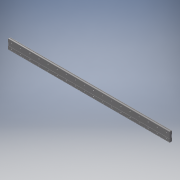
# Autodesk Inventor part: LWLF42...BCSR710Track Rail
Saved by Autodesk Inventor 2016 (Build 200138000, 138)
## iProperties
Category: PARTsolutions
Company: IKO
Created: 2015-04-20
Part Number: LWLF42...BCSR710Track Rail
Catalog Web Link: www.cadenas.de
Description: LWLF Track-LWLF
Vendor: IKO
Document SubType Name: Modeling
Designer: PARTuser1
Manufacturer: IKO
Mass: 2162.88 g
Surface Area: 840.251 cm^2
Volume: 270.361 cm^3
Density: 8 g/cm^3
Material: Stainless Steel
Appearance: Semi-Polished
PSOL_IDENT_0: {$CADENAS_DATA\23d-libs\iko\linear_way_series\linear_way_l_series\lwlf\lwlf4\lwlf_track.prj},207 {VT
PSOL_IDENT_1: YP=3D},{NB=LWLF42...BCSR710Track Rail},{LINA=LWLF42...BCSR710Track Rail},{NN=LWLF Track},{DATE=11.12
PSOL_IDENT_2: .2014 01:21:34},{GEOMDATE=16.10.2008 00:00:00},{VERSION=},{LINEID=230},{LINESUBID=-1},{WBVAR=L,SP,RE
PSOL_IDENT_3: F}  {NB=LWLF42...BCSR710Track Rail},{LINA=LWLF42...BCSR710Track Rail},{KT=DUMMY},{MN=LWLF42},{MNX=LW
PSOL_IDENT_4: LF42...BCS},{L=710.00},{SP=},{REF=},{W=42.000},{H4=10.000},{D3=4.500},{D4=8.000},{HM=4.500},{E1=15},
PSOL_IDENT_5: {E2=15},{F=40.000},{H1=4.000},{L1D=1075.00},{NX=1},{N=1},{N1=1},{P=18},{SP1='', 'No', 'S', 'Yes'},{P
PSOL_IDENT_6: 1D=53},{LS=1520.000},{LMAX=1600.000},{LX=680},{LY=1520},{LZ=1560},{PS=38},{LMINS=67},{EK=30},{EMIN=6
PSOL_IDENT_7: .500},{EMINJ=6.500},{EMAXJ=26.500},{PV=110},{P1D1=55},{EMIND=6.5},{LV=2230},{ED=20},{ED1=0},{L1=54.8
PSOL_IDENT_8: 00},{L4=60.000},{A=2.500},{C=2.000},{LMIN=60.00},{LEND=1560.00},{RK=1.50},{GC=7.76},{KX=21.20},{KY=7
PSOL_IDENT_9: .00},{RV=0.355},{RH=0.194},{MR=0.40},{GRX=0.40},{GRY=0.50},{GR=1.00},{LC=2.00},{IX=18.50},{IY=0.60}
SUPPLIER: IKO
ARTICLENO: LWLF42...BCSR710Track Rail
BOMINFO: LWLF42...BCSR710Track Rail
CREATOR: CADENAS GmbH
Title: LWLF42...BCSR710Track Rail
Author: Cadenas PARTsolutions
Comments: LWLF
Autodesk Inventor part; units mm, degrees
sketch "Sketch_1" plane through (-15, 0, 0) normal (1, 0, 0) x (0, 0, -1)
  line L0 (-21, 0.5) -> (-20.5, 0)
  line L1 (-20.5, 0) -> (20.5, 0)
  line L2 (20.5, 0) -> (21, 0.5)
  line L3 (21, 0.5) -> (21, 5.5134)
  arc A0 (19.9068, 6.24) -> (21, 5.5134) centre (21.2, 7) ccw
  line L4 (19.9068, 6.24) -> (19.194, 6.3657)
  arc A1 (19, 6.595) -> (19.194, 6.3657) centre (19.38, 6.7198) ccw
  line L5 (19, 6.595) -> (19, 7.405)
  arc A2 (19.194, 7.6343) -> (19, 7.405) centre (19.38, 7.2802) ccw
  line L6 (19.194, 7.6343) -> (19.9068, 7.76)
  arc A3 (21, 8.4866) -> (19.9068, 7.76) centre (21.2, 7) ccw
  line L7 (21, 8.4866) -> (21, 9.5)
  arc A4 (21, 9.5) -> (20.6, 10) centre (20.0602, 9.1582) ccw
  line L8 (20.6, 10) -> (-20.6, 10)
  arc A5 (-20.6, 10) -> (-21, 9.5) centre (-20.0602, 9.1582) ccw
  line L9 (-21, 9.5) -> (-21, 8.4866)
  arc A6 (-19.9068, 7.76) -> (-21, 8.4866) centre (-21.2, 7) ccw
  line L10 (-19.9068, 7.76) -> (-19.194, 7.6343)
  arc A7 (-19, 7.405) -> (-19.194, 7.6343) centre (-19.38, 7.2802) ccw
  line L11 (-19, 7.405) -> (-19, 6.595)
  arc A8 (-19.194, 6.3657) -> (-19, 6.595) centre (-19.38, 6.7198) ccw
  line L12 (-19.194, 6.3657) -> (-19.9068, 6.24)
  arc A9 (-21, 5.5134) -> (-19.9068, 6.24) centre (-21.2, 7) ccw
  line L13 (-21, 5.5134) -> (-21, 0.5)
  constraints: 28 end point, 20 point on circle, 10 centre point
extrude "Extrusion1" add sketch "Sketch_1" along normal blind 710
sketch "Sketch_24" plane through (-15, 0, 0) normal (1, 0, 0) x (0, 0, -1)
  line L0 (-42, -5) -> (42, -5)
  line L1 (42, -5) -> (42, 15)
  line L2 (42, 15) -> (-42, 15)
  line L3 (-42, 15) -> (-42, -5)
  line L4 (-21, 0) -> (-6.5, 0)
  line L5 (-6.5, 0) -> (-5.9, 0.6)
  line L6 (-5.9, 0.6) -> (5.9, 0.6)
  line L7 (5.9, 0.6) -> (6.5, 0)
  line L8 (6.5, 0) -> (21, 0)
  line L9 (21, 0) -> (21, 10)
  line L10 (21, 10) -> (6.5, 10)
  line L11 (6.5, 10) -> (5.9, 9.4)
  line L12 (5.9, 9.4) -> (-5.9, 9.4)
  line L13 (-5.9, 9.4) -> (-6.5, 10)
  line L14 (-6.5, 10) -> (-21, 10)
  line L15 (-21, 10) -> (-21, 0)
  constraints: 32 end point
extrude "Extrusion2" cut sketch "Sketch_24" along normal blind 710
sketch "Sketch_22" plane through (0, 0, 11.5) normal (0, 0, 1) x (1, 0, 0)
  line L0 (0, 0) -> (0, 10)
  line L1 (0, 10) -> (4, 10)
  line L2 (4, 10) -> (4, 5.5)
  line L3 (4, 5.5) -> (2.25, 5.5)
  line L4 (2.25, 5.5) -> (2.25, 0.2)
  line L5 (2.25, 0.2) -> (2.45, 0)
  line L6 (2.45, 0) -> (0, 0)
  line L7 (0, 0) -> (0, 10)
  constraints: 16 end point
revolve "Revolution1" cut sketch "Sketch_22" angle 360 about axis through (0, 0, 11.5) along (0, -1, 0)
pattern_linear "Rectangular Pattern1" count 18 spacing 40 along (1, 0, 0) of "Revolution1"
sketch "Sketch_2" plane through (0, 0, -11.5) normal (0, 0, 1) x (1, 0, 0)
  line L0 (0, 0) -> (0, 10)
  line L1 (0, 10) -> (4, 10)
  line L2 (4, 10) -> (4, 5.5)
  line L3 (4, 5.5) -> (2.25, 5.5)
  line L4 (2.25, 5.5) -> (2.25, 0.2)
  line L5 (2.25, 0.2) -> (2.45, 0)
  line L6 (2.45, 0) -> (0, 0)
  line L7 (0, 0) -> (0, 10)
  constraints: 16 end point
revolve "Revolution2" cut sketch "Sketch_2" angle 360 about axis through (0, 0, -11.5) along (0, -1, 0)
pattern_linear "Rectangular Pattern2" count 18 spacing 40 along (1, 0, 0) of "Revolution2"
sketch "Sketch_11" plane through (-15, 0, 0) normal (1, 0, 0) x (0, 0, -1)
  circle A0 centre (18.5, -0.6) radius 0.8
  constraints: 1 centre point
extrude "Extrusion3" cut sketch "Sketch_11" along normal blind 710
ref_plane "dummy_XY" through (0, 0, 0) normal (1, 0, 0) x (0, 0, -1)
ref_plane "dummy_YZ" through (0, 0, 0) normal (0, 0, -1) x (0, 1, 0)
ref_plane "dummy_ZX" through (0, 0, 0) normal (0, 1, 0) x (1, 0, 0)
ref_plane "pin_2_XY" through (692.5, 10, 0) normal (0, 0, 1) x (1, 0, 0)
ref_plane "pin_2_YZ" through (692.5, 10, 0) normal (1, 0, 0) x (0, 1, 0)
ref_plane "pin_2_ZX" through (692.5, 10, 0) normal (0, 1, 0) x (0, 0, 1)
ref_plane "slider_XY" through (-15, 4, 0) normal (1, 0, 0) x (0, 0, -1)
ref_plane "slider_YZ" through (-15, 4, 0) normal (0, 0, -1) x (0, 1, 0)
ref_plane "slider_ZX" through (-15, 4, 0) normal (0, 1, 0) x (1, 0, 0)
ref_plane "stop_pin_XY" through (-12.5, 10, 0) normal (0, 0, 1) x (1, 0, 0)
ref_plane "stop_pin_YZ" through (-12.5, 10, 0) normal (1, 0, 0) x (0, 1, 0)
ref_plane "stop_pin_ZX" through (-12.5, 10, 0) normal (0, 1, 0) x (0, 0, 1)
body "Solid1"
